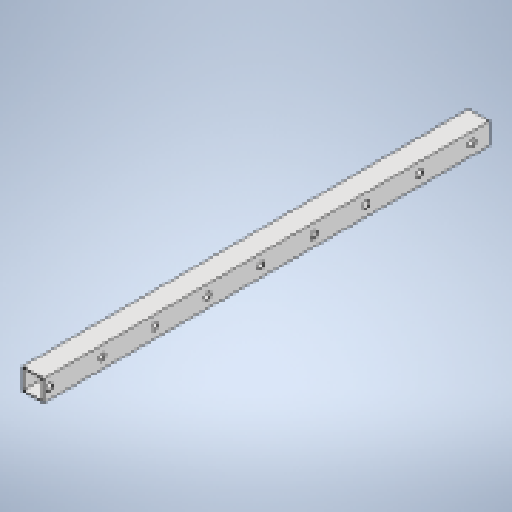
# Autodesk Inventor part: TKS 3534 FDS WAY tube4
Saved by Autodesk Inventor 2025 (Build 290162010, 162A)
## iProperties
Created: 2025-06-24
Part Number: TKS 3534 FDS WAY tube4
Material: Stainless Steel
Document SubType Name: Modeling
Designer: admin
Mass: 1762.25 g
Surface Area: 2283.33 cm^2
Volume: 220.281 cm^3
Density: 8 g/cm^3
Sheet Metal Rule: AISI304 2mm Die16
Sheet Metal Width: 0.000 mm
Sheet Metal Length: 0.000 mm
Sheet Metal Area: 0.000 mm^2
Appearance: Default
Author: user
Autodesk Inventor part; units mm, degrees
ref_plane "YZ Plane" through (0, 0, 0) normal (1, 0, 0) x (0, 1, 0)
ref_plane "XZ Plane" through (0, 0, 0) normal (0, 1, 0) x (-1, 0, 0)
ref_plane "XY Plane" through (0, 0, 0) normal (0, 0, 1) x (1, 0, 0)
sketch "Sketch9" plane through (0, 0, 0) normal (0, 1, 0) x (-1, 0, 0)
  line L0 (25, 25) -> (-25, 25)
  line L1 (-25, 25) -> (-25, -25)
  line L2 (-25, -25) -> (25, -25)
  line L3 (25, -25) -> (25, 25)
  line L4 (25, 25) -> (-25, -25) construction
  line L5 (-25, 25) -> (25, -25) construction
  line L6 (-23, 23) -> (23, 23)
  line L7 (23, 23) -> (23, -23)
  line L8 (23, -23) -> (-23, -23)
  line L9 (-23, -23) -> (-23, 23)
  point P0 (0, 0)
  dimension "d172" = 50
  dimension "d173" = 50
  dimension "d174" = 2
  constraints: 20 end point, 4 parallel, 2 midpoint, 2 perpendicular, 1 horizontal, 3 other
  measures "d172" distance of L2.end L1.end
  measures "d173" distance of L0.end L1.end
  measures "d174" distance between parallel lines of L0 L6
extrude "Extrusion3" add sketch "Sketch9" against normal blind 1055
sketch "Sketch10" plane through (0, 0, 0) normal (1, 0, 0) x (0, 1, 0)
  line L0 (0, 25) -> (0, -25) construction
  line L1 (0, 25) -> (-1055, 25) construction
  line L2 (-1055, -25) -> (-1055, 25) construction
  line L3 (0, -25) -> (-1055, -25) construction
  line L4 (-1050, 8.5) -> (-1033, 8.5)
  line L5 (-1033, 8.5) -> (-1033, -8.5)
  line L6 (-1033, -8.5) -> (-1050, -8.5)
  line L7 (-1050, -8.5) -> (-1050, 8.5)
  line L8 (-1050, 8.5) -> (-1033, -8.5) construction
  line L9 (-1033, 8.5) -> (-1050, -8.5) construction
  circle A0 centre (-1041.5, 0) radius 8.5
  line L10 (0, 25) -> (0, -25) projected
  point P0 (0, 0)
  point P1 (0, 0)
  point P2 (-1055, 0)
  dimension "d177" = 17
  dimension "d178" = 17
  dimension "d191" = 5
  constraints: 12 end point, 4 midpoint, 2 parallel, 1 centre point, 1 coincident, 1 horizontal, 1 horizontal alignment, 1 perpendicular, 1 tangent
  measures "d177" distance of L4.start L4.end
  measures "d178" distance of L4.end L5.end
  measures "d191" distance between parallel lines of L7 L2
extrude "Extrusion4" cut sketch "Sketch10" along normal through all contours A0
pattern_linear "Rectangular Pattern4" count 9 spacing 125 along (0, 1, 0) of "Extrusion4"
body "Solid4"
